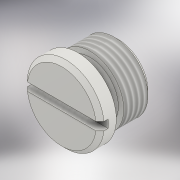
# Autodesk Inventor part: 螺塞
Saved by Autodesk Inventor 2020 (Build 240168000, 168)
## iProperties
Created: 2021-04-21
Part Number: 螺塞
Material: 钢 AISI 1018 106 HR
Document SubType Name: Modeling
Designer: Luorily
Density: 7.87 g/cm^3
Appearance: 钢
Author: Luorily
Autodesk Inventor part; units mm, degrees
ref_plane "YZ Plane" through (0, 0, 0) normal (1, 0, 0) x (0, 1, 0)
ref_plane "XZ Plane" through (0, 0, 0) normal (0, 1, 0) x (-1, 0, 0)
ref_plane "XY Plane" through (0, 0, 0) normal (0, 0, 1) x (1, 0, 0)
sketch "草图1" plane through (0, 0, 0) normal (0, 0, 1) x (1, 0, 0)
  circle A0 centre (0, 0) radius 9.5
  dimension "d0" = 19
  constraints: 1 centre point, 1 coincident
  measures "d0" diameter of A0
extrude "拉伸1" add sketch "草图1" along normal blind 4
sketch "草图2" plane through (0, 0, 0) normal (0, 0, -1) x (-1, 0, 0)
  circle A0 centre (0, 0) radius 9.5 projected
  circle A1 centre (0, 0) radius 7
  dimension "d3" = 14
  constraints: 1 centre point, 1 coincident
  measures "d3" diameter of A1
extrude "拉伸2" add sketch "草图2" along normal blind 3 contours A1
sketch "草图3" plane through (0, 0, -3) normal (0, 0, -1) x (-1, 0, 0)
  circle A0 centre (0, 0) radius 7 projected
  circle A1 centre (0, 0) radius 8.3315
  dimension "d6" = 14
  dimension "d7" = 16.663
  constraints: 1 centre point, 1 coincident
  measures "d6" diameter of A0
  measures "d7" diameter of A1
extrude "拉伸3" add sketch "草图3" along normal blind 7 contours A0 | A1
thread "螺纹1" size "G16.662x1.337" designation "G 3/8" class "A" standard "GB Pipe Threads without seal" length 22
chamfer "倒角1" distance 1 angle 45 2 edges at (8.3315, 0, -10) (-9.5, 0, 4)
sketch "草图4" plane through (0, 0, 4) normal (0, 0, 1) x (1, 0, 0)
  circle A0 centre (0, 0) radius 8.5 projected
  line L0 (0, 0) -> (0, 1)
  line L1 (0, 1) -> (21.5358, 1)
  line L2 (21.5358, 1) -> (-22.0631, 1)
  line L3 (-22.0631, 1) -> (-22.0631, -1)
  line L4 (-22.0631, -1) -> (21.5358, -1)
  line L5 (21.5358, -1) -> (21.5358, 1)
  dimension "d15" = 1
  dimension "d16" = 2
  constraints: 12 end point, 2 parallel, 2 perpendicular, 1 horizontal, 1 vertical
  measures "d15" distance of L0.start L0.end
  measures "d16" distance of L3.end L2.end
extrude "拉伸4" cut sketch "草图4" against normal blind 2 contours A0 L4 L2 L1 | A0 L1 L5 L4 | A0 L4 L3 L2
